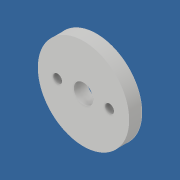
# Autodesk Inventor part: Handle Cover Plate
Saved by Autodesk Inventor 2018 (Build 220112000, 112)
## iProperties
Created: 2017-12-22
Part Number: Handle Cover Plate
Material: Generic
Document SubType Name: Modeling
Designer: 232963
Density: 1 g/cm^3
Appearance: Default
Author: 232963
Autodesk Inventor part; units mm, degrees
ref_plane "YZ Plane" through (0, 0, 0) normal (1, 0, 0) x (0, 1, 0)
ref_plane "XZ Plane" through (0, 0, 0) normal (0, 1, 0) x (-1, 0, 0)
ref_plane "XY Plane" through (0, 0, 0) normal (0, 0, 1) x (1, 0, 0)
sketch "Sketch1" plane through (0, 0, 0) normal (0, 0, 1) x (1, 0, 0)
  circle A0 centre (0, 0) radius 22.225
  circle A1 centre (-12.7, 0) radius 2.1844
  circle A2 centre (0, 0) radius 4.7625
  circle A3 centre (12.7, 0) radius 2.1844
  dimension "d0" = 44.45
  dimension "d1" = 4.3688
  dimension "d2" = 12.7
  dimension "d3" = 12.7
  dimension "d4" = 9.525
  constraints: 4 centre point, 2 coincident, 1 equal radius
  measures "d0" diameter of A0
  measures "d1" diameter of A1
  measures "d2" distance of point (0, 0) A1.centre
  measures "d3" distance of point (0, 0) A3.centre
  measures "d4" diameter of A2
extrude "Extrusion1" add sketch "Sketch1" along normal blind 6.35
body "Solid1"
